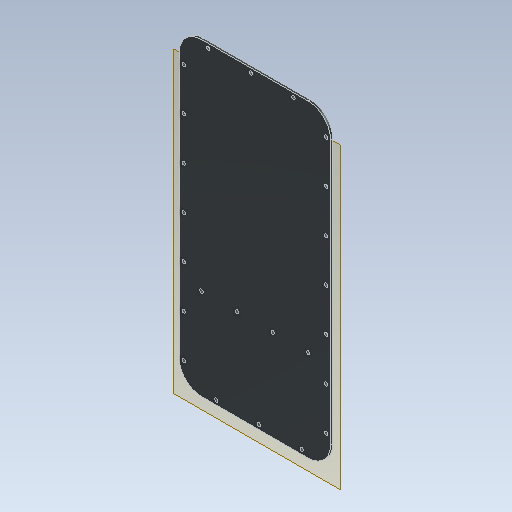
# Autodesk Inventor part: Крышка фонаря 2
Saved by Autodesk Inventor 2021 (Build 250183000, 183)
## iProperties
Created: 2020-12-11
Part Number: Крышка фонаря 2
Material: Чугун, серый
Document SubType Name: Modeling
Designer: Тимоха
Mass: 7294.7 g
Surface Area: 4201.82 cm^2
Volume: 1020.24 cm^3
Density: 7.15 g/cm^3
Appearance: Чугун серый
Author: Тимоха
Autodesk Inventor part; units mm, degrees
ref_plane "YZ Plane" through (0, 0, 0) normal (1, 0, 0) x (0, 1, 0)
ref_plane "XZ Plane" through (0, 0, 0) normal (0, 1, 0) x (-1, 0, 0)
ref_plane "XY Plane" through (0, 0, 0) normal (0, 0, 1) x (1, 0, 0)
ref_plane "РабПлоскость1" through (0, 0, 0) normal (0, 0, 1) x (1, 0, 0)
sketch "Эскиз1" plane through (0, 0, 0) normal (0, 0, 1) x (1, 0, 0)
  circle A0 centre (120, -100) radius 4 projected
  circle A1 centre (40, -100) radius 4 projected
  circle A2 centre (-40, -100) radius 4 projected
  circle A3 centre (-120, -100) radius 4 projected
  circle A4 centre (-86.7655, -295) radius 4 projected
  circle A5 centre (9.3009, -295) radius 4 projected
  circle A6 centre (105.3673, -295) radius 4 projected
  circle A7 centre (160, -236.3982) radius 4 projected
  circle A8 centre (160, -140.3319) radius 4 projected
  circle A9 centre (160, -44.2655) radius 4 projected
  circle A10 centre (160, 51.8009) radius 4 projected
  circle A11 centre (160, 147.8673) radius 4 projected
  circle A12 centre (160, 243.9336) radius 4 projected
  circle A13 centre (160, 340) radius 4 projected
  circle A14 centre (86.7655, 380) radius 4 projected
  circle A15 centre (-9.3009, 380) radius 4 projected
  circle A16 centre (-105.3673, 380) radius 4 projected
  circle A17 centre (-160, 321.3982) radius 4 projected
  circle A18 centre (-160, 225.3319) radius 4 projected
  circle A19 centre (-160, 129.2655) radius 4 projected
  circle A20 centre (-160, 33.1991) radius 4 projected
  circle A21 centre (-160, -62.8673) radius 4 projected
  circle A22 centre (-160, -158.9336) radius 4 projected
  circle A23 centre (-160, -255) radius 4 projected
  line L0 (170, -255) -> (170, 340) projected
  arc A24 (170, 340) -> (120, 390) centre (120, 340) ccw projected
  line L1 (120, 390) -> (-120, 390) projected
  arc A25 (-120, 390) -> (-170, 340) centre (-120, 340) ccw projected
  line L2 (-170, 340) -> (-170, -255) projected
  arc A26 (-170, -255) -> (-120, -305) centre (-120, -255) ccw projected
  line L3 (-120, -305) -> (120, -305) projected
  arc A27 (120, -305) -> (170, -255) centre (120, -255) ccw projected
  line L4 (-120, -120) -> (120, -120) projected
  arc A28 (150, -150) -> (120, -120) centre (120, -150) ccw projected
  line L5 (150, -150) -> (150, -255) projected
  arc A29 (120, -285) -> (150, -255) centre (120, -255) ccw projected
  line L6 (120, -285) -> (-120, -285) projected
  arc A30 (-150, -255) -> (-120, -285) centre (-120, -255) ccw projected
  line L7 (-150, -255) -> (-150, -150) projected
  arc A31 (-120, -120) -> (-150, -150) centre (-120, -150) ccw projected
  line L8 (150, 340) -> (150, -50) projected
  arc A32 (120, -80) -> (150, -50) centre (120, -50) ccw projected
  line L9 (120, -80) -> (-120, -80) projected
  arc A33 (-150, -50) -> (-120, -80) centre (-120, -50) ccw projected
  line L10 (-150, -50) -> (-150, 340) projected
  arc A34 (-120, 370) -> (-150, 340) centre (-120, 340) ccw projected
  line L11 (-120, 370) -> (120, 370) projected
  arc A35 (150, 340) -> (120, 370) centre (120, 340) ccw projected
  point P0 (0, 0)
extrude "Выдавливание1" add sketch "Эскиз1" along normal blind 5 contours A27 L3 A26 L2 A25 L1 A24 L0 | L4 A28 L5 A29 L6 A30 L7 A31 | L8 A32 L9 A33 L10 A34 L11 A35
